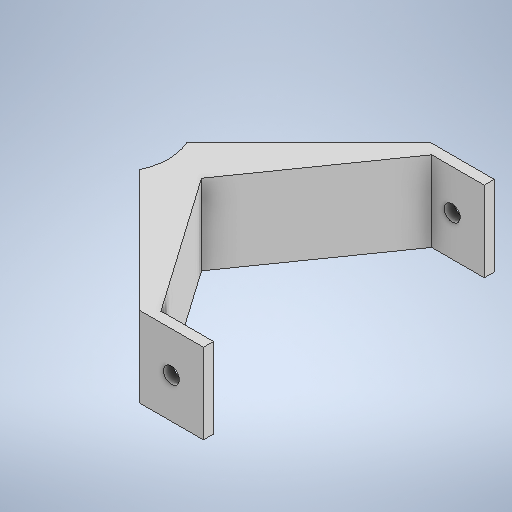
# Autodesk Inventor part: NeckRest
Saved by Autodesk Inventor 2025.1 (Build 291241000, 241)
## iProperties
Created: 2025-12-01
Part Number: NeckRest
Material: Generic
Document SubType Name: Modeling
Designer: Juxin
Density: 1 g/cm^3
Appearance: Default
Author: Juxin
Title: Neck Rest
Autodesk Inventor part; units mm, degrees
ref_plane "YZ Plane" through (0, 0, 0) normal (1, 0, 0) x (0, 1, 0)
ref_plane "XZ Plane" through (0, 0, 0) normal (0, 1, 0) x (-1, 0, 0)
ref_plane "XY Plane" through (0, 0, 0) normal (0, 0, 1) x (1, 0, 0)
sketch "Sketch1" plane through (0, 0, 0) normal (0, 1, 0) x (-1, 0, 0)
  line L0 (0, 0) -> (0, -46.0375)
  line L1 (0, 0) -> (20.32, 0)
  line L2 (16.6421, -3.175) -> (0, -3.175)
  line L3 (0, -3.175) -> (0, 0)
  line L4 (0, -46.0375) -> (57.15, -46.0375)
  line L5 (0, -46.0375) -> (57.15, -46.0375) construction
  line L6 (20.32, 0) -> (59.69, 0) construction
  line L7 (20.32, -3.175) -> (52.07, -3.175) construction
  arc A0 (75.1105, -28.077) -> (57.15, -46.0375) centre (75.1105, -46.0375) ccw
  line L8 (57.15, -46.0375) -> (75.1105, -28.077) construction
  line L9 (57.15, -46.0375) -> (82.55, -46.0375) construction
  line L10 (20.32, 0) -> (58.8119, -38.4919)
  line L11 (20.32, 0) -> (74.7558, 0) construction
  line L12 (20.32, -3.175) -> (72.6455, -3.175) construction
  line L13 (0, -92.075) -> (0, -46.0375)
  line L14 (16.6421, -3.175) -> (46.6548, -46.0375)
  line L15 (16.6421, -3.175) -> (68.9676, -3.175) construction
  line L16 (0, -92.075) -> (0, -46.0375)
  line L17 (0, -92.075) -> (20.32, -92.075)
  line L18 (16.6421, -88.9) -> (0, -88.9)
  line L19 (0, -88.9) -> (0, -92.075)
  line L20 (20.32, -92.075) -> (59.69, -92.075) construction
  line L21 (20.32, -88.9) -> (52.07, -88.9) construction
  arc A1 (57.15, -46.0375) -> (75.1105, -63.998) centre (75.1105, -46.0375) ccw
  line L22 (57.15, -46.0375) -> (75.1105, -63.998) construction
  line L23 (20.32, -92.075) -> (58.8119, -53.5831)
  line L24 (20.32, -92.075) -> (74.7558, -92.075) construction
  line L25 (20.32, -88.9) -> (72.6455, -88.9) construction
  line L26 (16.6421, -88.9) -> (46.6548, -46.0375)
  line L27 (16.6421, -88.9) -> (68.9676, -88.9) construction
  dimension "d1" = 20.32
  dimension "d6" = 0
  dimension "d26" = 25.4
  dimension "d27" = 45
  dimension "d29" = 45
  dimension "d31" = 55
  dimension "d34" = 92.075
  constraints: 56 end point, 12 symmetric about line, 9 horizontal, 6 point on circle, 4 equal length, 2 centre point, 1 line through centre, 1 parallel, 1 point on line, 1 vertical, 1 other
  measures "d1" distance of L7.start L2.end
  measures "d6" distance between parallel lines of L4 L5
  measures "d26" distance of L5.end L8.end
  measures "d27" angle of L9 L8
  measures "d29" angle of L10 L11
  measures "d31" angle of L14 L15
  measures "d34" distance of L13.start L0.start
extrude "Extrusion1" add sketch "Sketch1" along normal blind 25.4 contours L1 L10 A0 L4 L14 L2 L0 | L4 A1 L23 L17 L13 L18 L26
sketch "Sketch2" plane through (-20.32, 0, 0) normal (0, 0, 1) x (1, 0, 0)
  line L0 (20.32, 0) -> (20.32, 25.4) projected
  line L1 (20.32, 12.7) -> (10.16, 12.7)
  circle A0 centre (10.16, 12.7) radius 2.54
  dimension "d19" = 10.16
  dimension "d20" = 5.08
  constraints: 2 end point, 1 centre point, 1 coincident, 1 horizontal, 1 midpoint
  measures "d19" distance of L1.start L1.end
  measures "d20" diameter of A0
extrude "Extrusion2" cut sketch "Sketch2" against normal blind 142.875
body "Solid1"
